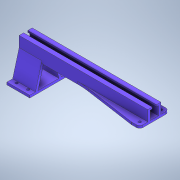
# Autodesk Inventor part: reyka
Saved by Autodesk Inventor 2020 (Build 240168000, 168)
## iProperties
Created: 2022-07-27
Part Number: reyka
Material: Типовые
Document SubType Name: Modeling
Designer: akapu
Density: 1 g/cm^3
Appearance: По умолчанию
Author: akapu
Autodesk Inventor part; units mm, degrees
ref_plane "YZ Plane" through (0, 0, 0) normal (1, 0, 0) x (0, 1, 0)
ref_plane "XZ Plane" through (0, 0, 0) normal (0, 1, 0) x (-1, 0, 0)
ref_plane "XY Plane" through (0, 0, 0) normal (0, 0, 1) x (1, 0, 0)
sketch "Эскиз2" plane through (0, 0, 0) normal (1, 0, 0) x (0, 1, 0)
  line L0 (0, 0) -> (-3, 0)
  line L1 (-3, 0) -> (-3, 36)
  line L2 (-3, 36) -> (0, 36)
  line L3 (0, 36) -> (0, 0)
  line L4 (-3, 0) -> (0, 0)
  line L5 (0, 0) -> (0, -5)
  line L6 (0, -5) -> (-3, -5)
  line L7 (-3, -5) -> (-3, 0)
  line L8 (-3, 36) -> (0, 36)
  line L9 (0, 36) -> (0, 41)
  line L10 (0, 41) -> (-3, 41)
  line L11 (-3, 41) -> (-3, 36)
  line L12 (0, 0) -> (0, 36)
  line L13 (0, 36) -> (0, 34)
  line L14 (0, 0) -> (0, 2)
  line L15 (29.146, 18) -> (29.146, 26)
  line L16 (29.146, 26) -> (29.146, 10)
  line L17 (29.146, 10) -> (0, 2)
  line L18 (29.146, 26) -> (0, 34)
  point P0 (19.146, 0)
  dimension "d4" = 3
  dimension "d5" = 36
  dimension "d6" = 5
  dimension "d7" = 5
  dimension "d8" = 19.146
  dimension "d13" = 2
  dimension "d14" = 2
  constraints: 38 end point, 6 parallel, 6 point on line, 3 horizontal, 3 perpendicular
  measures "d4" distance of L1.end L2.end
  measures "d5" distance of L0.end L1.end
  measures "d6" distance of L4.end L5.end
  measures "d7" distance of L9.end L8.end
  measures "d8" distance of point (19.146, 0) L12.start
  measures "d13" distance of L8.end L13.end
  measures "d14" distance of L12.start L14.end
extrude "Выдавливание2" add sketch "Эскиз2" along normal blind 3
sketch "Эскиз3" plane through (3, 0, 0) normal (1, 0, 0) x (0, 0, -1)
  line L0 (5, -3) -> (5, 0) projected
  line L1 (5, 0) -> (-41, 0) projected
  line L2 (5, -3) -> (-41, -3)
  line L3 (-41, -3) -> (-41, 0)
  line L4 (-41, 0) -> (5, 0)
  line L5 (5, 0) -> (5, -3)
  point P0 (0, 0)
  point P1 (-34, 0)
  constraints: 8 end point, 2 parallel, 1 horizontal, 1 perpendicular
extrude "Выдавливание3" add sketch "Эскиз3" along normal blind 25
sketch "Эскиз5" plane through (0, 0, 2) normal (0, 1, 0) x (1, 0, 0)
  line L0 (0, 7) -> (28, 7) projected
  line L1 (0, 7) -> (0, 2)
  line L2 (0, 7) -> (0, 0) projected
  line L3 (0, 2) -> (28, 2)
  line L4 (28, -39) -> (28, 7) projected
  line L5 (0, 7) -> (0, -39) projected
  line L6 (0, -39) -> (0, -34)
  line L7 (0, -34) -> (28, -34)
  line L8 (28, -34) -> (21, -34)
  line L9 (21, -34) -> (7, -34)
  line L10 (7, -34) -> (7, 2)
  circle A0 centre (7, -34) radius 1.6
  circle A1 centre (21, -34) radius 1.6
  circle A2 centre (7, 2) radius 1.6
  circle A3 centre (21, 2) radius 1.6
  point P0 (0, -32)
  dimension "d17" = 5
  dimension "d18" = 7
  dimension "d19" = 14
  dimension "d20" = 3.2
  dimension "d21" = 3.2
  dimension "d22" = 3.2
  dimension "d23" = 3.2
  constraints: 14 end point, 6 point on line, 4 centre point, 3 coincident, 3 perpendicular, 1 collinear
  measures "d17" distance of L5.end L6.end
  measures "d18" distance of L7.end L8.end
  measures "d19" distance of L8.end L9.end
  measures "d20" diameter of A0
  measures "d21" diameter of A1
  measures "d22" diameter of A2
  measures "d23" diameter of A3
extrude "Выдавливание4" cut sketch "Эскиз5" against normal blind 25 contours A2 L3 | L3 L10 A2 | A3 L3 | L3 A3 | L3 A2 L10 | A1 L7 | L7 A1 | A0 L10 L7 | L7 A0 | A0 L7 L10
sketch "Эскиз7" plane through (3, 0, 0) normal (1, 0, 0) x (0, 0, -1)
  line L0 (-10, 29.146) -> (-26, 29.146) projected
  line L1 (-26, 29.146) -> (-10, 29.146)
  line L2 (-10, 29.146) -> (-10, 26.146)
  line L3 (-10, 26.146) -> (-26, 26.146)
  line L4 (-26, 26.146) -> (-26, 29.146)
  point P0 (0, 0)
  dimension "d37" = 3
  constraints: 8 end point, 2 parallel, 1 horizontal, 1 perpendicular
  measures "d37" distance of L1.end L2.end
extrude "Выдавливание6" add sketch "Эскиз7" along normal blind 155 and the other way blind 3
sketch "Эскиз8" plane through (0, 29.146, 26) normal (0, 1, 0) x (1, 0, 0)
  line L0 (158, 16) -> (158, 0) projected
  line L1 (0, -15) -> (0, 31) projected
  line L2 (158, 16) -> (0, 16)
  line L3 (0, 16) -> (0, 13)
  line L4 (0, 13) -> (158, 13)
  line L5 (158, 13) -> (158, 16)
  line L6 (0, 0) -> (3, 0) projected
  line L7 (0, 0) -> (158, 0)
  line L8 (158, 0) -> (158, 3)
  line L9 (158, 3) -> (0, 3)
  line L10 (0, 3) -> (0, 0)
  point P0 (0, 26)
  point P1 (158, 3)
  point P2 (0, 3)
  dimension "d38" = 3
  dimension "d39" = 3
  constraints: 16 end point, 4 parallel, 2 horizontal, 2 perpendicular, 2 point on line
  measures "d38" distance of L3.end L2.end
  measures "d39" distance of L8.end L7.end
extrude "Выдавливание7" add sketch "Эскиз8" along normal blind 11 contours L0 L4 L1 L2 | L0 L7 L6 L1 L9
sketch "Эскиз9" plane through (3, 0, 0) normal (1, 0, 0) x (0, 0, -1)
  line L0 (-26, 29.146) -> (-34, 0) projected
  line L1 (-34, 0) -> (-26, 29.146)
  line L2 (-26, 29.146) -> (-10, 29.146)
  line L3 (-10, 29.146) -> (-2.177, 0)
  line L4 (-2.177, 0) -> (-34, 0)
  line L5 (-1.6, 0) -> (1.6, 0) projected
  line L6 (-26, 29.146) -> (-23.107, 28.3519)
  line L7 (-23.107, 28.3519) -> (-30.889, 0)
  line L8 (-2, 0) -> (-10, 29.146) projected
  line L9 (-2, 0) -> (-5.111, 0)
  line L10 (-34, 0) -> (-2, 0) projected
  line L11 (-10, 29.146) -> (-12.8975, 28.3685)
  line L12 (-10, 29.146) -> (-7, 29.146) construction
  line L13 (-12.8975, 28.3685) -> (-5.111, 0)
  point P0 (0, 0)
  dimension "d42" = 3
  dimension "d43" = 3.111
  dimension "d44" = 3
  dimension "d45" = 164.98
  constraints: 20 end point, 2 collinear, 2 horizontal, 2 perpendicular, 1 equal length, 1 point on line
  measures "d42" distance of L0.start L6.end
  measures "d43" distance of L8.start L9.end
  measures "d44" distance of L2.end L11.end
  measures "d45" angle of L11 L12
extrude "Выдавливание8" add sketch "Эскиз9" along normal blind 25 contours L6 L7 L4 L0 | L3 L4 L13 L11
sketch "Эскиз10" plane through (0, 40.146, 26) normal (0, 1, 0) x (1, 0, 0)
  line L0 (0, 0) -> (0, -8) projected
  line L1 (158, 16) -> (28, 16) projected
  line L2 (0, 0) -> (158, 0)
  line L3 (158, 0) -> (158, 16)
  line L4 (158, 16) -> (0, 16)
  line L5 (0, 16) -> (0, 0)
  line L6 (0, -15) -> (0, 31) projected
  line L7 (0, 8) -> (0, 10.5)
  line L8 (0, 10.5) -> (0, 5.5)
  line L9 (0, 5.5) -> (158, 5.5)
  line L10 (158, 13) -> (158, 3) projected
  line L11 (158, 5.5) -> (158, 10.5)
  line L12 (158, 10.5) -> (0, 10.5)
  line L13 (0, 13) -> (158, 13) projected
  point P0 (0, 26)
  point P1 (28, 16)
  dimension "d48" = 2.5
  dimension "d49" = 5
  constraints: 18 end point, 4 point on line, 3 parallel, 2 perpendicular, 1 horizontal, 1 midpoint
  measures "d48" distance of L7.start L7.end
  measures "d49" distance of L7.end L8.end
extrude "Выдавливание9" add sketch "Эскиз10" along normal blind 2 contours L3 L13 L5 L4 L1 | L3 L12 L5 L13 | L3 L2 L5 L9
sketch "Эскиз11" plane through (28, 26.146, 10) normal (0, -1, 0) x (1, 0, 0)
  line L0 (130, 0) -> (-28, 0) projected
  line L1 (130, 0) -> (130, -10)
  line L2 (125, -5) -> (125, 21)
  line L3 (130, 16) -> (130, 10.5) projected
  line L4 (130, 21) -> (130, 16)
  line L5 (130, 16) -> (130, 21)
  line L6 (130, 21) -> (130, 26)
  line L7 (130, 26) -> (120, 26)
  line L8 (120, 26) -> (120, -10)
  line L9 (120, -10) -> (130, -10)
  line L10 (-28, 16) -> (130, 16) projected
  line L11 (51, 16) -> (120, 26)
  line L12 (120, -10) -> (51, 0)
  circle A0 centre (125, 21) radius 1.6
  circle A1 centre (125, -5) radius 1.6
  point P0 (-28, -10)
  dimension "d52" = 10
  dimension "d54" = 26
  dimension "d56" = 10
  dimension "d57" = 3.2
  dimension "d58" = 3.2
  constraints: 20 end point, 3 perpendicular, 2 centre point, 2 coincident, 2 collinear, 2 midpoint, 1 point on line, 1 vertical
  measures "d52" distance of L0.start L1.end
  measures "d54" distance of L2.start L2.end
  measures "d56" distance of L6.end L7.end
  measures "d57" diameter of A0
  measures "d58" diameter of A1
extrude "Выдавливание10" add sketch "Эскиз11" against normal blind 3 contours L1 L9 L8 L0 | L8 L12 L0 | L10 L8 L7 L6 L4 | L10 L11 L8
fillet "Сопряжение1" radius 4 4 edges at (158, 27.646, 36) (158, 27.646, 0) (148, 27.646, 0) (148, 27.646, 36)
fillet "Сопряжение2" radius 100 2 edges at (79, 27.646, 10) (79, 27.646, 26)
